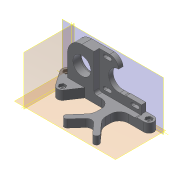
# Autodesk Inventor part: Cycl_marcoFrontalY
Saved by Autodesk Inventor 2015 SP2 (Build 190223200, 223)
## iProperties
Created: 2015-04-21
Material: Genérico
Document SubType Name: Modeling
Designer: E.Beroiz
Density: 1 g/cm^3
Appearance: Valor por defecto
Description: Cycl_marcoFrontalY
Author: E.Beroiz
Autodesk Inventor part; units mm, degrees
sketch "Boceto2" plane through (0, 0, 0) normal (0, 0, 1) x (1, 0, 0)
  line L0 (0, 0) -> (91.459, 0)
  arc A0 (91.459, -11) -> (91.459, 0) centre (91.459, -5.5) ccw
  line L1 (91.459, -11) -> (74, -11)
  arc A1 (74, -11) -> (64, -21) centre (74, -21) ccw
  line L2 (64, -21) -> (64, -26)
  line L3 (54, -26) -> (54, -21)
  line L4 (54, -26) -> (64, -26) construction
  arc A2 (50.8805, -34.1233) -> (54, -26) centre (41.8635, -26) ccw
  arc A3 (64, -26) -> (67.1195, -34.1233) centre (76.1365, -26) ccw
  line L5 (50.8805, -34.1233) -> (40.3387, -45.8251)
  line L6 (67.1195, -34.1233) -> (77.6613, -45.8251)
  arc A4 (40.3387, -45.8251) -> (44.7965, -49.841) centre (42.5676, -47.833) ccw
  line L7 (44.7965, -49.841) -> (54.5422, -39.023)
  arc A5 (63.4578, -39.023) -> (54.5422, -39.023) centre (59, -43.039) ccw
  line L8 (63.4578, -39.023) -> (73.2035, -49.841)
  arc A6 (73.2035, -49.841) -> (77.6613, -45.8251) centre (75.4324, -47.833) ccw
  circle A7 centre (0, -5.5) radius 1.88
  circle A8 centre (91.459, -5.5) radius 1.88
  arc A9 (0, 0) -> (-4.5119, -8.6452) centre (0, -5.5) ccw
  line L9 (-4.5119, -8.6452) -> (6.9893, -25.1441)
  arc A10 (6.9893, -25.1441) -> (16.0775, -25.0498) centre (11.5012, -21.9989) ccw
  line L10 (16.0775, -25.0498) -> (25.444, -11)
  arc A11 (54, -21) -> (44, -11) centre (44, -21) ccw
  line L11 (25.444, -11) -> (44, -11)
  circle A12 centre (11.5012, -21.9989) radius 1.88
  point P0 (59, -26)
  dimension "d19" = 91.459
  dimension "d20" = 5.5
  dimension "d21" = 5
  dimension "d22" = 5
  dimension "d25" = 10
  dimension "d28" = 84.03
  dimension "d29" = 15.75
  dimension "d31" = 3
  dimension "d32" = 3
  dimension "d34" = 6
  dimension "d35" = 3.76
  dimension "d36" = 3.76
  dimension "d37" = 10
  dimension "d38" = 5.5
  dimension "d39" = 5.5
  dimension "d40" = 91.459
  dimension "d41" = 5.5
  dimension "d42" = 68.57
  dimension "d43" = 123.69
  dimension "d44" = 20.112
  dimension "d46" = 3.76
  constraints: 24 end point, 20 point on circle, 18 tangent, 13 centre point, 6 horizontal alignment, 3 horizontal, 3 parallel, 2 coincident, 2 vertical, 1 equal length, 1 equal radius, 1 midpoint, 1 vertical alignment
  measures "d19" distance of L0.start L0.end
  measures "d20" radius of A0
  measures "d21" distance of L2.start L2.end
  measures "d22" distance of L3.start L3.end
  measures "d25" distance between parallel lines of L3 L2
  measures "d28" angle of L6 L5
  measures "d29" distance of L6.start L6.end
  measures "d31" radius of A6
  measures "d32" radius of A4
  measures "d34" radius of A5
  measures "d35" diameter of A7
  measures "d36" diameter of A8
  measures "d37" radius of A11
  measures "d38" radius of A9
  measures "d39" distance from line of L0 A7.centre
  measures "d40" distance of A0.centre A7.centre
  measures "d41" radius of A10
  measures "d42" angle of L10 L9
  measures "d43" angle of L10 L11
  measures "d44" distance of L9.start L9.end
  measures "d46" diameter of A12
extrude "Extrusión1" add sketch "Boceto2" along normal blind 10
sketch "Boceto4" plane through (0, 0, 10) normal (0, 0, 1) x (1, 0, 0)
  circle A0 centre (0, -5.5) radius 1.88 projected
  circle A1 centre (11.5012, -21.9989) radius 1.88 projected
  circle A2 centre (91.459, -5.5) radius 1.88 projected
  line L0 (1.7999, -2.3825) -> (3.5998, -5.5)
  line L1 (3.5998, -5.5) -> (1.7999, -8.6175)
  line L2 (1.7999, -8.6175) -> (-1.7999, -8.6175)
  line L3 (-1.7999, -8.6175) -> (-3.5998, -5.5)
  line L4 (-3.5998, -5.5) -> (-1.7999, -2.3825)
  line L5 (-1.7999, -2.3825) -> (1.7999, -2.3825)
  line L6 (13.3011, -18.8814) -> (15.101, -21.9989)
  line L7 (15.101, -21.9989) -> (13.3011, -25.1164)
  line L8 (13.3011, -25.1164) -> (9.7013, -25.1164)
  line L9 (9.7013, -25.1164) -> (7.9015, -21.9989)
  line L10 (7.9015, -21.9989) -> (9.7013, -18.8814)
  line L11 (9.7013, -18.8814) -> (13.3011, -18.8814)
  line L12 (89.6591, -2.3825) -> (93.2589, -2.3825)
  line L13 (93.2589, -2.3825) -> (95.0588, -5.5)
  line L14 (95.0588, -5.5) -> (93.2589, -8.6175)
  line L15 (93.2589, -8.6175) -> (89.6591, -8.6175)
  line L16 (89.6591, -8.6175) -> (87.8592, -5.5)
  line L17 (87.8592, -5.5) -> (89.6591, -2.3825)
  point P0 (0, 0)
  dimension "d49" = 6.235
  dimension "d50" = 6.235
  dimension "d51" = 6.235
  constraints: 36 end point, 3 coincident, 3 horizontal, 39 other
  measures "d49" distance between parallel lines of L2 L5
  measures "d50" distance between parallel lines of L15 L12
  measures "d51" distance between parallel lines of L8 L11
extrude "Extrusión2" cut sketch "Boceto4" against normal blind 2.79
sketch "Boceto5" plane through (0, 0, 10) normal (0, 0, 1) x (1, 0, 0)
  line L0 (87.8592, -5.5) -> (89.6591, -2.3825) projected
  line L1 (89.6591, -2.3825) -> (93.2589, -2.3825) projected
  line L2 (93.2589, -2.3825) -> (95.0588, -5.5) projected
  line L3 (95.0588, -5.5) -> (93.2589, -8.6175) projected
  line L4 (93.2589, -8.6175) -> (89.6591, -8.6175) projected
  line L5 (89.6591, -8.6175) -> (87.8592, -5.5) projected
  line L6 (-1.7999, -2.3825) -> (1.7999, -2.3825) projected
  line L7 (1.7999, -2.3825) -> (3.5998, -5.5) projected
  line L8 (3.5998, -5.5) -> (1.7999, -8.6175) projected
  line L9 (1.7999, -8.6175) -> (-1.7999, -8.6175) projected
  line L10 (-1.7999, -8.6175) -> (-3.5998, -5.5) projected
  line L11 (-3.5998, -5.5) -> (-1.7999, -2.3825) projected
  line L12 (9.7013, -18.8814) -> (13.3011, -18.8814) projected
  line L13 (13.3011, -18.8814) -> (15.101, -21.9989) projected
  line L14 (15.101, -21.9989) -> (13.3011, -25.1164) projected
  line L15 (13.3011, -25.1164) -> (9.7013, -25.1164) projected
  line L16 (9.7013, -25.1164) -> (7.9015, -21.9989) projected
  line L17 (7.9015, -21.9989) -> (9.7013, -18.8814) projected
  line L18 (91.459, 0) -> (0, 0) projected
  arc A0 (0, 0) -> (-4.5119, -8.6452) centre (0, -5.5) ccw projected
  line L19 (-4.5119, -8.6452) -> (6.9893, -25.1441) projected
  arc A1 (6.9893, -25.1441) -> (16.0775, -25.0498) centre (11.5012, -21.9989) ccw projected
  line L20 (16.0775, -25.0498) -> (25.444, -11) projected
  line L21 (25.444, -11) -> (44, -11) projected
  arc A2 (54, -21) -> (44, -11) centre (44, -21) ccw projected
  line L22 (54, -21) -> (54, -26) projected
  arc A3 (50.8805, -34.1233) -> (54, -26) centre (41.8635, -26) ccw projected
  line L23 (50.8805, -34.1233) -> (40.3387, -45.8251) projected
  arc A4 (40.3387, -45.8251) -> (44.7965, -49.841) centre (42.5676, -47.833) ccw projected
  line L24 (44.7965, -49.841) -> (54.5422, -39.023) projected
  arc A5 (63.4578, -39.023) -> (54.5422, -39.023) centre (59, -43.039) ccw projected
  line L25 (63.4578, -39.023) -> (73.2035, -49.841) projected
  arc A6 (73.2035, -49.841) -> (77.6613, -45.8251) centre (75.4324, -47.833) ccw projected
  line L26 (77.6613, -45.8251) -> (67.1195, -34.1233) projected
  arc A7 (64, -26) -> (67.1195, -34.1233) centre (76.1365, -26) ccw projected
  line L27 (64, -26) -> (64, -21) projected
  arc A8 (74, -11) -> (64, -21) centre (74, -21) ccw projected
  line L28 (74, -11) -> (91.459, -11) projected
  arc A9 (91.459, -11) -> (91.459, 0) centre (91.459, -5.5) ccw projected
  line L29 (6.247, 0) -> (82.707, 0)
  line L30 (82.707, 0) -> (82.707, -11)
  line L31 (82.707, -11) -> (6.247, -11)
  line L32 (6.247, -11) -> (6.247, 0)
  dimension "d54" = 76.46
  dimension "d55" = 11
  dimension "d56" = 6.247
  constraints: 8 end point, 2 parallel, 1 horizontal, 1 perpendicular, 1 point on line
  measures "d54" distance of L30.end L31.end
  measures "d55" distance of L29.end L30.end
  measures "d56" distance from line of A0.centre L32
extrude "Extrusión3" add sketch "Boceto5" along normal blind 40 contours L30 L28 L31 L21 L32 L18
sketch "Boceto6" plane through (25.444, -11, 0) normal (0, -1, 0) x (1, 0, 0)
  circle A0 centre (-3.197, 29.5) radius 10
  line L0 (-19.197, 10) -> (-19.197, 50) projected
  line L1 (0, 10) -> (-19.197, 10) projected
  point P0 (-25.444, 0)
  point P1 (-3.197, 19.5)
  point P2 (-13.197, 29.5)
  dimension "d59" = 20
  dimension "d60" = 6
  dimension "d61" = 9.5
  constraints: 2 point on circle, 1 centre point, 1 horizontal alignment, 1 vertical alignment
  measures "d59" diameter of A0
  measures "d60" distance from line of L0 A0.end
  measures "d61" distance from line of L1 A0.start
extrude "Extrusión4" cut sketch "Boceto6" against normal through all
sketch "Boceto7" plane through (0, 0, 0) normal (0, 1, 0) x (1, 0, 0)
  circle A0 centre (22.247, -29.5) radius 10 projected
  circle A1 centre (22.247, -29.5) radius 11.3
  point P0 (0, 0)
  dimension "d64" = 22.6
  constraints: 1 centre point, 1 coincident
  measures "d64" diameter of A1
extrude "Extrusión5" cut sketch "Boceto7" against normal blind 3
chamfer "Chaflán2" [suppressed]
chamfer "Chaflán3" distance 0.8 angle 30 1 edges at (10.947, 0, 29.5) measured on face at (33.5104, -2, 30.4093)
sketch "Boceto8" plane through (25.444, -11, 0) normal (0, -1, 0) x (1, 0, 0)
  circle A0 centre (-3.197, 29.5) radius 11.7619 projected
  line L0 (57.263, 50) -> (-19.197, 50) projected
  line L1 (57.263, 10) -> (57.263, 50) projected
  line L2 (66.015, 10) -> (57.263, 10) projected
  line L3 (66.015, 0) -> (66.015, 10) projected
  line L4 (-25.444, 0) -> (66.015, 0) projected
  line L5 (-25.444, 0) -> (-25.444, 10) projected
  line L6 (-19.197, 10) -> (-25.444, 10) projected
  line L7 (-19.197, 10) -> (-19.197, 50) projected
  line L8 (66.015, 10) -> (57.263, 10) projected
  arc A1 (55.763, 8.85) -> (58.763, 11.85) centre (55.763, 11.85) ccw
  line L9 (55.763, 8.85) -> (13.263, 8.85)
  arc A2 (10.263, 11.85) -> (13.263, 8.85) centre (13.263, 11.85) ccw
  line L10 (58.763, 11.85) -> (58.763, 10)
  line L11 (10.263, 11.85) -> (10.263, 49.825)
  line L12 (10.263, 49.825) -> (10.263, 54.6666)
  line L13 (10.263, 54.6666) -> (60.2602, 54.6666)
  line L14 (60.2602, 54.6666) -> (58.763, 10)
  dimension "d77" = 1.5
  dimension "d78" = 3
  dimension "d79" = 1.15
  dimension "d80" = 48.5
  dimension "d82" = 40.975
  constraints: 12 end point, 4 point on circle, 3 horizontal alignment, 2 centre point, 2 tangent, 1 parallel, 1 perpendicular, 1 point on line, 1 vertical
  measures "d77" horizontal distance of L1.start L10.start
  measures "d78" radius of A2
  measures "d79" distance between parallel lines of L2 L9
  measures "d80" distance of L11.start L10.start
  measures "d82" distance from line of L9 L11.end
extrude "Extrusión6" cut sketch "Boceto8" against normal blind 6 contours L1 L2 A1 L9 A2 L11 L12 L0 | L0 L12 L13 L14 L10 A1 L2 L1
sketch "Boceto9" plane through (25.444, -11, 0) normal (0, 1, 0) x (1, 0, 0)
  line L0 (52.9884, -8.85) -> (52.9884, -17.0753)
  line L1 (52.2173, -10) -> (41.6755, -10) projected
  line L2 (14.1236, -10) -> (19.3525, -10) projected
  line L3 (14.1236, -8.85) -> (14.1236, -17.0753)
  line L4 (14.1236, -17.0753) -> (52.9884, -17.0753)
  line L5 (14.1236, -8.85) -> (52.9884, -8.85)
  line L6 (55.763, -8.85) -> (13.263, -8.85) projected
  point P0 (-25.444, 0)
  point P1 (14.8947, -10)
  constraints: 8 end point, 1 collinear, 1 horizontal alignment, 1 vertical
extrude "Extrusión7" cut sketch "Boceto9" against normal through all
sketch "Boceto10" plane through (25.444, -5, 0) normal (0, -1, 0) x (1, 0, 0)
  line L0 (10.263, 11.85) -> (10.263, 50) projected
  line L1 (57.263, 50) -> (57.263, 10) projected
  line L2 (10.263, 50) -> (57.263, 50) projected
  line L3 (10.263, 11.85) -> (10.263, 50) projected
  arc A0 (10.263, 11.85) -> (13.263, 8.85) centre (13.263, 11.85) ccw projected
  line L4 (55.763, 8.85) -> (13.263, 8.85) projected
  arc A1 (55.763, 8.85) -> (58.1247, 10) centre (55.763, 11.85) ccw projected
  arc A2 (31.763, 40.65) -> (33.018, 18.4209) centre (31.763, 29.5) ccw
  line L5 (33.018, 18.4209) -> (40.018, 18.4209)
  line L6 (31.763, 40.65) -> (57.263, 40.65)
  line L7 (40.018, 18.9209) -> (57.263, 18.9209)
  line L8 (57.263, 50) -> (57.263, 10) projected
  line L9 (40.018, 18.4209) -> (40.018, 18.9209)
  line L10 (57.263, 40.65) -> (57.263, 18.9209)
  circle A3 centre (-3.197, 29.5) radius 10 projected
  line L11 (57.263, 10) -> (58.1247, 10) projected
  point P0 (-25.444, 0)
  point P1 (10.263, 45)
  dimension "d87" = 22.3
  dimension "d88" = 7
  dimension "d90" = 17.245
  dimension "d91" = 0.5
  dimension "d109" = 25.5
  constraints: 10 end point, 3 horizontal, 2 point on circle, 2 vertical alignment, 1 centre point, 1 collinear, 1 horizontal alignment, 1 point on line, 1 tangent, 1 vertical
  measures "d87" diameter of A2
  measures "d88" distance of L5.start L5.end
  measures "d90" distance of L7.start L7.end
  measures "d91" distance between parallel lines of L5 L7
  measures "d109" distance from line of L8 A2.centre
extrude "Extrusión8" cut sketch "Boceto10" against normal blind 6 contours L1 L7 L9 L5 A2 L6
fillet "Empalme2" radius 4 1 edges at (65.462, -2.5, 18.4209)
sketch "Boceto12" plane through (25.444, -5, 0) normal (0, -1, 0) x (1, 0, 0)
  line L0 (10.263, 50) -> (57.263, 50) projected
  line L1 (10.263, 11.85) -> (10.263, 50) projected
  arc A0 (10.263, 11.85) -> (13.263, 8.85) centre (13.263, 11.85) ccw projected
  line L2 (55.763, 8.85) -> (13.263, 8.85) projected
  arc A1 (55.763, 8.85) -> (58.1247, 10) centre (55.763, 11.85) ccw projected
  line L3 (57.263, 18.9209) -> (57.263, 10) projected
  line L4 (57.263, 18.9209) -> (40.018, 18.9209) projected
  arc A2 (38.0815, 18.4209) -> (40.018, 18.9209) centre (38.0815, 22.4209) ccw projected
  line L5 (38.0815, 18.4209) -> (33.018, 18.4209) projected
  arc A3 (31.763, 40.65) -> (33.018, 18.4209) centre (31.763, 29.5) ccw projected
  line L6 (16.263, 16.4) -> (22.263, 16.4)
  arc A4 (22.263, 12.6) -> (22.263, 16.4) centre (22.263, 14.5) ccw
  line L7 (22.263, 12.6) -> (16.263, 12.6)
  arc A5 (16.263, 16.4) -> (16.263, 12.6) centre (16.263, 14.5) ccw
  line L8 (31.763, 40.65) -> (57.263, 40.65) projected
  line L9 (57.263, 50) -> (57.263, 40.65) projected
  line L10 (57.263, 10) -> (58.1247, 10) projected
  point P0 (-25.444, 0)
  dimension "d98" = 3.8
  dimension "d99" = 6
  dimension "d111" = 6
  dimension "d112" = 5.65
  constraints: 4 end point, 4 point on circle, 4 tangent, 2 centre point, 1 horizontal, 1 parallel
  measures "d98" distance between parallel lines of L7 L6
  measures "d99" distance of A5.centre A4.centre
  measures "d111" distance from line of L1 A5.centre
  measures "d112" distance from line of L2 A4.centre
extrude "Extrusión10" cut sketch "Boceto12" against normal blind 6 contours L6 A4 L7 A5
pattern_linear "Patrón rectangular1" count 2 spacing 31 along (0, 0, 1) of "Extrusión10"
pattern_linear "Patrón rectangular2" count 2 spacing 31 along (1, 0, 0) of "Extrusión10", "Patrón rectangular1"
fillet "Empalme3" radius 16 1 edges at (6.247, -5.5, 50)
sketch "Boceto13" plane through (0, 0, 0) normal (0, 1, 0) x (1, 0, 0)
  line L0 (82.707, -50) -> (22.247, -50) projected
  line L1 (82.707, -40.65) -> (82.707, -50) projected
  line L2 (82.707, -40.65) -> (57.207, -40.65) projected
  arc A0 (47.2281, -50) -> (57.207, -40.65) centre (47.2281, -40) ccw
  point P0 (0, 0)
  dimension "d114" = 10
  constraints: 2 point on circle, 1 centre point, 1 point on line, 1 tangent
  measures "d114" radius of A0
extrude "Extrusión11" cut sketch "Boceto13" against normal blind 10
